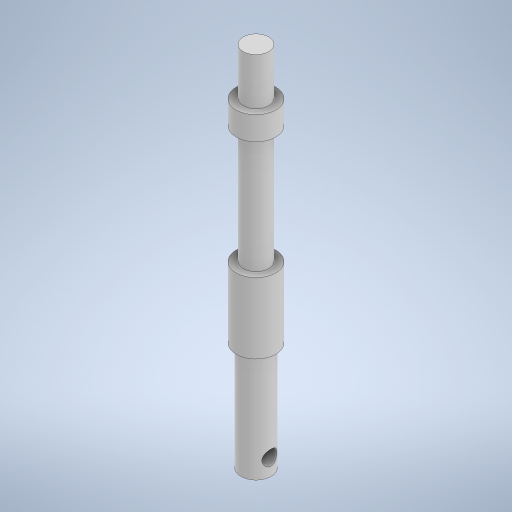
# Autodesk Inventor part: Valve
Saved by Autodesk Inventor 2023 (Build 270158000, 158)
## iProperties
Created: 2023-02-23
Part Number: Valve
Material: Generic
Document SubType Name: Modeling
Designer: tommy
Density: 1 g/cm^3
Appearance: Default
Author: tommy
Autodesk Inventor part; units mm, degrees
ref_plane "YZ Plane" through (0, 0, 0) normal (1, 0, 0) x (0, 1, 0)
ref_plane "XZ Plane" through (0, 0, 0) normal (0, 1, 0) x (-1, 0, 0)
ref_plane "XY Plane" through (0, 0, 0) normal (0, 0, 1) x (1, 0, 0)
sketch "Sketch1" plane through (0, 0, 0) normal (1, 0, 0) x (0, 1, 0)
  line L0 (19.812, -0.0127) -> (0, -0.0127)
  line L1 (5.842, -0.8255) -> (5.842, -1.0795)
  line L2 (0, -0.0127) -> (0, -0.8255)
  line L3 (5.842, -0.8255) -> (0, -0.8255)
  line L4 (5.842, -1.0795) -> (9.652, -1.0795)
  line L5 (5.842, -1.0795) -> (9.652, -1.0795)
  line L6 (16.002, -1.0795) -> (17.272, -1.0795)
  line L7 (9.652, -1.0795) -> (9.652, -0.6985)
  line L8 (19.812, -0.6985) -> (17.272, -0.6985)
  line L9 (16.002, -0.6985) -> (9.652, -0.6985)
  line L10 (17.272, -1.0795) -> (17.272, -0.6985)
  line L11 (16.002, -0.6985) -> (16.002, -1.0795)
  line L12 (19.812, -0.0127) -> (19.812, -0.6985)
  line L13 (16.637, -1.0795) -> (16.637, -0.0127)
  line L14 (16.637, -0.0127) -> (0.889, -0.0127)
  circle A0 centre (0.889, -0.0127) radius 0.3969
  dimension "d9" = 0.8128
  dimension "d10" = 1.0668
  dimension "d11" = 0.6858
  dimension "d12" = 1.0668
  dimension "d13" = 0.6858
  dimension "d14" = 1.27
  dimension "d15" = 6.35
  dimension "d16" = 3.81
  dimension "d17" = 5.842
  dimension "d18" = 2.54
  dimension "d20" = 15.748
  dimension "d21" = 0.7937
  constraints: 30 end point, 2 point on line, 1 centre point, 1 coincident, 1 midpoint, 1 perpendicular, 1 vertical
  measures "d9" distance between parallel lines of L0 L3
  measures "d10" distance between parallel lines of L0 L4
  measures "d11" distance between parallel lines of L0 L9
  measures "d12" distance between parallel lines of L0 L6
  measures "d13" distance between parallel lines of L0 L8
  measures "d14" distance of L6.start L6.end
  measures "d15" distance of L9.start L7.end
  measures "d16" distance of L1.end L4.end
  measures "d17" distance of L1.start L2.end
  measures "d18" distance of L8.start L8.end
  measures "d20" distance of L13.end L14.end
  measures "d21" diameter of A0
revolve "Revolution1" add sketch "Sketch1" angle 360 about axis through (0, 19.812, -0.0127) along (0, -1, 0) picked at (1.1498, -0.0444) contours L12 L8 L10 L6 L13 L0 | L13 L6 L11 L9 L7 L4 L1 L3 L2 L0 A0 | A0 L0
extrude "Extrusion1" cut sketch "Sketch1" along normal mid plane 25.4 contours A0 L0 | L0 A0
body "Solid1"
